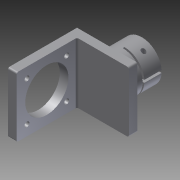
# Autodesk Inventor part: zweifach nema v2
Saved by Autodesk Inventor 2011 (Build 150239000, 239)
## iProperties
Created: 2015-05-27
Part Number: zweifach nema v2
Document SubType Name: Modeling
Designer: schmieder
Density: 1 g/cm^3
Author: schmieder
Autodesk Inventor part; units mm, degrees
ref_plane "Arbeitsebene10" through (-35, 70.3553, 70.3553) normal (0, 1, 0) x (1, 0, 0)
sketch "Skizze7" plane through (-35, 70.3553, 70.3553) normal (0, 1, 0) x (1, 0, 0)
  circle A0 centre (17.5, 17.2929) radius 11.5
  point P0 (35, 70.3553)
  dimension "d32" = 23
  constraints: 1 centre point
  measures "d32" diameter of A0
extrude "Achshalter" add sketch "Skizze7" along normal blind 20
ref_plane "Arbeitsebene11" through (-17.5, 90.3553, 53.0624) normal (0, 1, 0) x (1, 0, 0)
sketch "Skizze16" plane through (-17.5, 90.3553, 53.0624) normal (0, 1, 0) x (1, 0, 0)
  circle A0 centre (0, 0) radius 11.5 projected
  arc A1 (2.2, 1.3856) -> (2.2, -1.3856) centre (0, 0) ccw
  line L0 (2.2, 1.3856) -> (2.2, -1.3856)
  point P0 (17.5, 53.0624)
  dimension "d54" = 5.2
  dimension "d55" = 2.2
  constraints: 2 end point, 2 point on circle, 1 centre point, 1 coincident, 1 vertical
  measures "d54" diameter of A1
  measures "d55" distance from line of L0 A0.centre
extrude "Extrusion11" cut sketch "Skizze16" against normal blind 18 contours L0 A1
ref_plane "Arbeitsebene2" through (-35, 80.3553, 35.7696) normal (0, 1, 0) x (1, 0, 0)
sketch "Skizze17" plane through (-35, 80.3553, 35.7696) normal (0, 1, 0) x (1, 0, 0)
  line L0 (30.7802, -4.1446) -> (17.4658, -4.1446)
  line L1 (17.4658, -4.1446) -> (17.4658, -31.1746)
  line L2 (17.4658, -31.1746) -> (30.7802, -31.1746)
  line L3 (30.7802, -31.1746) -> (30.7802, -4.1446)
  point P0 (35, 35.7696)
  constraints: 8 end point, 2 parallel, 1 horizontal, 1 perpendicular
extrude "Extrusion12" cut sketch "Skizze17" against normal blind 1
ref_plane "Arbeitsebene16" through (-34, 67.3553, 52.8553) normal (0, 0, 1) x (1, 0, 0)
sketch "Skizze18" plane through (-34, 67.3553, 52.8553) normal (0, 0, 1) x (1, 0, 0)
  line L0 (29.7456, 25.5785) -> (16.4577, 25.5785)
  line L1 (16.4577, 25.5785) -> (16.4577, 12.5204)
  line L2 (16.4577, 12.5204) -> (29.7456, 12.5204)
  line L3 (29.7456, 12.5204) -> (29.7456, 25.5785)
  point P0 (34, -67.3553)
  constraints: 8 end point, 2 parallel, 1 horizontal, 1 perpendicular
extrude "Extrusion13" cut sketch "Skizze18" along normal blind 1 and the other way blind 0.5
ref_plane "Arbeitsebene17" through (-34, 67.3553, 70.3553) normal (0, 0, 1) x (1, 0, 0)
sketch "Skizze19" plane through (-34, 67.3553, 70.3553) normal (0, 0, 1) x (1, 0, 0)
  circle A0 centre (22.3096, 18.1328) radius 1.25
  point P0 (34, -67.3553)
  dimension "d67" = 2.5
  constraints: 1 centre point
  measures "d67" diameter of A0
extrude "Extrusion14" cut sketch "Skizze19" against normal blind 35
sketch "Skizze24" plane through (-17.5, 70.3553, 53.0624) normal (0, -1, 0) x (1, 0, 0)
  line L0 (-17.5, 17.5) -> (17.5, 17.5)
  line L1 (17.5, 17.5) -> (17.5, -17.5)
  line L2 (17.5, -17.5) -> (-17.5, -17.5)
  line L3 (-17.5, -17.5) -> (-17.5, 17.5)
  point P0 (0, 0)
  point P1 (17.5, -53.0624)
  dimension "d90" = 35
  dimension "d91" = 35
  dimension "d92" = 17.5
  dimension "d93" = 17.5
  constraints: 8 end point, 2 parallel, 1 horizontal, 1 perpendicular
  measures "d90" distance of L0.start L0.end
  measures "d91" distance of L0.end L1.end
  measures "d92" distance from line of L0 point (0, 0)
  measures "d93" distance from line of point (0, 0) L1
extrude "Extrusion17" add sketch "Skizze24" along normal blind 5
sketch "Skizze25" plane through (-35, 70.3553, 35.5624) normal (-1, 0, 0) x (0, 0, 1)
  line L0 (35, -5) -> (0, -5)
  line L1 (0, -5) -> (0, -40)
  line L2 (0, -40) -> (35, -40)
  line L3 (35, -40) -> (35, -5)
  point P0 (-35.5624, -70.3553)
  dimension "d96" = 35
  dimension "d97" = 35
  constraints: 8 end point, 2 parallel, 1 horizontal, 1 perpendicular
  measures "d96" distance of L2.end L1.end
  measures "d97" distance of L1.end L0.end
extrude "Extrusion18" add sketch "Skizze25" against normal blind 5
fillet "Rundung14" radius 1 1 edges at (-30, 65.3553, 53.0624)
fillet "Rundung15" radius 1 4 edges at (0, 67.8553, 70.5624) (0, 67.8553, 35.5624) (-32.5, 30.3553, 35.5624) (-32.5, 30.3553, 70.5624)
sketch "Skizze26" plane through (-35, 70.3553, 35.5624) normal (-1, 0, 0) x (0, 0, 1)
  line L0 (1, -40) -> (34, -40) projected
  circle A0 centre (17.5, -22.5) radius 12.5
  point P0 (-35.5624, -70.3553)
  dimension "d102" = 25
  dimension "d103" = 17.5
  constraints: 1 centre point
  measures "d102" diameter of A0
  measures "d103" distance from line of L0 A0.centre
extrude "Extrusion19" cut sketch "Skizze26" against normal up to surface (5 mm away)
sketch "Skizze27" plane through (-35, 70.3553, 35.5624) normal (-1, 0, 0) x (0, 0, 1)
  circle A0 centre (29, -34) radius 1.4
  circle A1 centre (29, -11) radius 1.4
  circle A2 centre (6, -11) radius 1.4
  circle A3 centre (6, -34) radius 1.4
  point P0 (-35.5624, -70.3553)
  dimension "d106" = 2.8
  dimension "d107" = 2.8
  dimension "d108" = 2.8
  dimension "d109" = 2.8
  dimension "d110" = 23
  dimension "d111" = 23
  dimension "d112" = 23
  dimension "d113" = 23
  constraints: 4 centre point
  measures "d106" diameter of A0
  measures "d107" diameter of A1
  measures "d108" diameter of A2
  measures "d109" diameter of A3
  measures "d110" distance of A0.centre A1.centre
  measures "d111" distance of A2.centre A1.centre
  measures "d112" distance of A3.centre A2.centre
  measures "d113" distance of A3.centre A0.centre
extrude "Extrusion20" cut sketch "Skizze27" against normal up to surface (5 mm away)
sketch "Skizze28" plane through (-35, 70.3553, 35.5624) normal (-1, 0, 0) x (0, 0, 1)
  circle A0 centre (29, -34) radius 1.4 projected
  circle A1 centre (29, -11) radius 1.4 projected
  circle A2 centre (6, -34) radius 1.4 projected
  circle A3 centre (6, -11) radius 1.4 projected
  circle A4 centre (29, -11) radius 2.5
  circle A5 centre (29, -34) radius 2.5
  circle A6 centre (6, -11) radius 2.5
  circle A7 centre (6, -34) radius 2.5
  point P0 (-35.5624, -70.3553)
  dimension "d116" = 5
  dimension "d117" = 5
  dimension "d118" = 5
  dimension "d119" = 5
  constraints: 4 centre point, 4 coincident
  measures "d116" diameter of A4
  measures "d117" diameter of A5
  measures "d118" diameter of A6
  measures "d119" diameter of A7
extrude "Extrusion21" cut sketch "Skizze28" against normal blind 2
